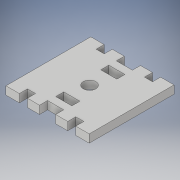
# Autodesk Inventor part: part_plunger_handle_side1
Saved by Autodesk Inventor 2017 (Build 210142000, 142)
## iProperties
Created: 2017-01-19
Part Number: part_plunger_handle_side1
Material: Generic
Document SubType Name: Modeling
Designer: John
Density: 1 g/cm^3
Appearance: Default
Author: John
Autodesk Inventor part; units mm, degrees
ref_plane "YZ Plane" through (0, 0, 0) normal (1, 0, 0) x (0, 1, 0)
ref_plane "XZ Plane" through (0, 0, 0) normal (0, 1, 0) x (-1, 0, 0)
ref_plane "XY Plane" through (0, 0, 0) normal (0, 0, 1) x (1, 0, 0)
sketch "Sketch2" plane through (0, 0, 0) normal (0, 1, 0) x (-1, 0, 0)
  line L0 (15.3786, -15.8442) -> (10.3786, -15.8442)
  line L1 (-15.6214, -15.8442) -> (-15.6214, -0.0442)
  line L2 (2.8786, -7.0442) -> (-3.1214, -7.0442)
  line L3 (-3.1214, -7.0442) -> (-3.1214, -10.0442)
  line L4 (-3.1214, -10.0442) -> (2.8786, -10.0442)
  line L5 (2.8786, -10.0442) -> (2.8786, -7.0442)
  line L6 (2.8786, -7.0442) -> (-3.1214, -10.0442) construction
  line L7 (-3.1214, -7.0442) -> (2.8786, -10.0442) construction
  line L8 (-3.1214, -15.8442) -> (-7.6214, -15.8442)
  line L9 (-3.1214, -12.8442) -> (2.8786, -12.8442)
  line L10 (2.8786, -12.8442) -> (2.8786, -15.8442)
  line L11 (-3.1214, -12.8442) -> (-3.1214, -15.8442)
  line L12 (15.3786, -0.0442) -> (15.3786, -15.8442)
  line L13 (10.3786, -15.8442) -> (10.3786, -12.8442)
  line L14 (10.3786, -12.8442) -> (7.3786, -12.8442)
  line L15 (7.3786, -12.8442) -> (7.3786, -15.8442)
  line L16 (7.3786, -15.8442) -> (2.8786, -15.8442)
  line L17 (-7.6214, -15.8442) -> (-7.6214, -12.8442)
  line L18 (-7.6214, -12.8442) -> (-10.6214, -12.8442)
  line L19 (-10.6214, -12.8442) -> (-10.6214, -15.8442)
  line L20 (-10.6214, -15.8442) -> (-15.6214, -15.8442)
  line L21 (-15.6214, 15.7558) -> (-15.6214, -0.0442)
  line L22 (15.3786, -0.0442) -> (15.3786, 15.7558)
  line L23 (2.6375, 6.9558) -> (2.6375, 9.9558)
  line L24 (2.6375, 9.9558) -> (-3.3625, 9.9558)
  line L25 (-3.3625, 9.9558) -> (-3.3625, 6.9558)
  line L26 (-3.3625, 6.9558) -> (2.6375, 6.9558)
  line L27 (15.3786, -0.0442) -> (-15.6214, -0.0442) construction
  line L28 (15.3786, 15.7558) -> (10.3786, 15.7558)
  line L29 (10.3786, 15.7558) -> (10.3786, 12.7558)
  line L30 (10.3786, 12.7558) -> (7.3786, 12.7558)
  line L31 (7.3786, 12.7558) -> (7.3786, 15.7558)
  line L32 (7.3786, 15.7558) -> (2.8786, 15.7558)
  line L33 (2.8786, 15.7558) -> (2.8786, 12.7558)
  line L34 (2.8786, 12.7558) -> (-3.1214, 12.7558)
  line L35 (-3.1214, 12.7558) -> (-3.1214, 15.7558)
  line L36 (-3.1214, 15.7558) -> (-7.6214, 15.7558)
  line L37 (-7.6214, 15.7558) -> (-7.6214, 12.7558)
  line L38 (-7.6214, 12.7558) -> (-10.6214, 12.7558)
  line L39 (-10.6214, 12.7558) -> (-10.6214, 15.7558)
  line L40 (-10.6214, 15.7558) -> (-15.6214, 15.7558)
  circle A0 centre (0, 0) radius 2.35
  point P0 (-0.1214, -8.5442)
  dimension "d3" = 3
  dimension "d11" = 6
  dimension "d12" = 15.8
  dimension "d13" = 3
  dimension "d14" = 3
  dimension "d15" = 4.5
  dimension "d479" = 6
  dimension "d485" = 31
  dimension "d486" = 5
  dimension "d493" = 7
  dimension "d494" = 7
  dimension "d497" = 4.7
  constraints: 82 end point, 21 equal length, 16 perpendicular, 11 parallel, 10 point on line, 4 horizontal, 2 midpoint, 1 centre point, 1 coincident, 1 collinear, 1 vertical, 2 other
  measures "d3" distance of L3.end L2.end
  measures "d11" distance of L9.start L9.end
  measures "d12" distance of L12.start L0.start
  measures "d13" distance of L15.end L0.end
  measures "d14" distance of L13.end L0.end
  measures "d15" distance of L15.end L10.end
  measures "d479" distance of L2.start L2.end
  measures "d485" distance of L12.start L1.end
  measures "d486" distance between parallel lines of L13 L12
  measures "d493" distance between parallel lines of L27 L2
  measures "d494" distance between parallel lines of L27 L26
  measures "d497" diameter of A0
extrude "Extrusion4" add sketch "Sketch2" along normal blind 3
body "Solid4"
